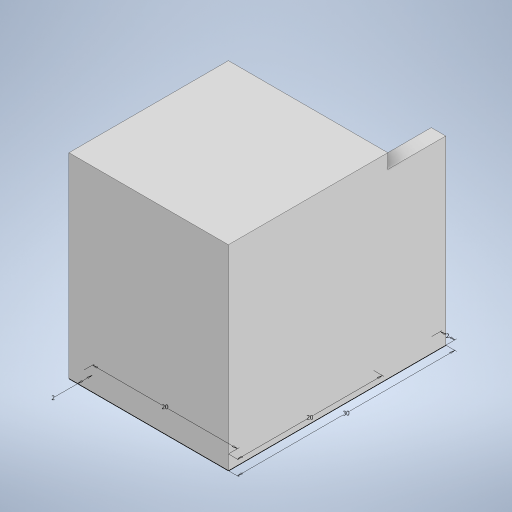
# Autodesk Inventor part: LaptopHalt
Saved by Autodesk Inventor 2023.1 (Build 271208000, 208)
## iProperties
Created: 2022-09-21
Part Number: LaptopHalt
Material: Generisch
Document SubType Name: Modeling
Designer: schwa
Density: 1 g/cm^3
Appearance: Vorgabe
Author: schwa
Autodesk Inventor part; units mm, degrees
ref_plane "YZ Plane" through (0, 0, 0) normal (1, 0, 0) x (0, 1, 0)
ref_plane "XZ Plane" through (0, 0, 0) normal (0, 1, 0) x (-1, 0, 0)
ref_plane "XY Plane" through (0, 0, 0) normal (0, 0, 1) x (1, 0, 0)
sketch "Skizze1" plane through (0, 0, 0) normal (0, 1, 0) x (-1, 0, 0)
  line L0 (0, 0) -> (-2, 0)
  line L1 (-2, 0) -> (-2, -30)
  line L2 (-2, -30) -> (0, -30)
  line L3 (0, -30) -> (0, 0)
  line L4 (0, 0) -> (20, 0)
  line L5 (20, 0) -> (20, -2)
  line L6 (20, -2) -> (0, -2)
  line L7 (0, -2) -> (0, 0)
  line L8 (20, -2) -> (0, -2)
  line L9 (0, -2) -> (0, -22)
  line L10 (0, -22) -> (20, -22)
  line L11 (20, -22) -> (20, -2)
  point P0 (0, -2)
  dimension "d0" = 2
  dimension "d1" = 30
  dimension "d2" = 20
  dimension "d3" = 2
  dimension "d4" = 20
  constraints: 24 end point, 6 parallel, 3 horizontal, 3 perpendicular, 1 point on line
  measures "d0" distance of L2.end L1.end
  measures "d1" distance of L1.end L0.end
  measures "d2" distance of L5.end L6.end
  measures "d3" distance between parallel lines of L4 L6
  measures "d4" distance of L9.end L8.end
extrude "Extrusion1" add sketch "Skizze1" along normal blind 2 contours L6 L11 L10 L3
extrude "Extrusion2" add sketch "Skizze1" along normal blind 25 contours L3 L2 L1 L0 | L4 L5 L6 L3
sketch "Skizze2" plane through (0, 25, 0) normal (0, 1, 0) x (1, 0, 0)
  line L0 (2, 0) -> (2, 30) projected
  line L1 (-20, 22) -> (-20, 0) projected
  line L2 (2, 0) -> (-20, 0)
  line L3 (-20, 0) -> (-20, 22)
  line L4 (-20, 22) -> (2, 22)
  line L5 (2, 22) -> (2, 0)
  point P0 (0, 0)
  constraints: 8 end point, 2 parallel, 1 horizontal, 1 perpendicular
extrude "Extrusion3" add sketch "Skizze2" along normal blind 2
